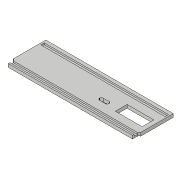
# Autodesk Inventor part: Electronics Container Part 4
Saved by Autodesk Inventor 2018.3 (Build 223284000, 284)
## iProperties
Created: 2019-03-04
Part Number: Electronics Container Part 4
Material: Generic
Document SubType Name: Modeling
Designer: aye06091
Mass: 12.6073 g
Surface Area: 108.421 cm^2
Volume: 12.6073 cm^3
Density: 1 g/cm^3
Appearance: Default
Author: aye06091
Autodesk Inventor part; units mm, degrees
ref_plane "YZ Plane" through (0, 0, 0) normal (1, 0, 0) x (0, 1, 0)
ref_plane "XZ Plane" through (0, 0, 0) normal (0, 1, 0) x (-1, 0, 0)
ref_plane "XY Plane" through (0, 0, 0) normal (0, 0, 1) x (1, 0, 0)
sketch "Sketch1" plane through (0, 0, 0) normal (0, 1, 0) x (-1, 0, 0)
  line L0 (0, 0) -> (-123.825, 0)
  line L1 (-123.825, 0) -> (-123.825, 38.1)
  line L2 (-123.825, 38.1) -> (0, 38.1)
  line L3 (0, 38.1) -> (0, 0)
  dimension "d0" = 123.825
  dimension "d1" = 38.1
  constraints: 8 end point, 2 parallel, 1 horizontal, 1 perpendicular
  measures "d0" distance of L0.start L0.end
  measures "d1" distance of L0.end L1.end
extrude "Extrusion1" add sketch "Sketch1" along normal blind 3.175
sketch "Sketch2" plane through (0, 3.175, 0) normal (0, 1, 0) x (1, 0, 0)
  line L0 (123.825, 0) -> (0, 0) projected
  line L1 (0, 0) -> (0, -38.1) projected
  line L2 (0, -38.1) -> (123.825, -38.1) projected
  line L3 (123.825, -38.1) -> (123.825, 0) projected
  line L4 (0, -36.5125) -> (123.825, -36.5125)
  line L5 (123.825, -36.5125) -> (123.825, -33.3121)
  line L6 (123.825, -33.3121) -> (0, -33.3121)
  line L7 (0, -33.3121) -> (0, -36.5125)
  line L8 (1.5875, -3.175) -> (122.2375, -3.175)
  line L9 (122.2375, -3.175) -> (122.2375, -6.604)
  line L10 (122.2375, -6.604) -> (1.5875, -6.604)
  line L11 (1.5875, -6.604) -> (1.5875, -3.175)
  dimension "d6" = 3.2004
  dimension "d7" = 1.5875
  dimension "d10" = 3.175
  dimension "d11" = 3.429
  dimension "d12" = 1.5875
  dimension "d13" = 1.5875
  constraints: 16 end point, 4 parallel, 2 horizontal, 2 perpendicular, 2 point on line
  measures "d6" distance between parallel lines of L4 L6
  measures "d7" distance between parallel lines of L2 L4
  measures "d10" distance between parallel lines of L0 L8
  measures "d11" distance between parallel lines of L10 L8
  measures "d12" distance between parallel lines of L1 L11
  measures "d13" distance between parallel lines of L3 L9
extrude "Extrusion2" cut sketch "Sketch2" against normal blind 1.5875 contours L3 L4 L1 L6
sketch "Sketch3" plane through (0, 3.175, 0) normal (0, 1, 0) x (1, 0, 0)
  line L0 (123.825, -33.3121) -> (123.825, 0) projected
  line L1 (123.825, 0) -> (0, 0) projected
  line L2 (0, 0) -> (0, -33.3121) projected
  line L3 (1.5875, -3.175) -> (122.2375, -3.175)
  line L4 (122.2375, -3.175) -> (122.2375, -6.604)
  line L5 (122.2375, -6.604) -> (1.5875, -6.604)
  line L6 (1.5875, -6.604) -> (1.5875, -3.175)
  dimension "d14" = 1.5875
  dimension "d15" = 1.5875
  dimension "d16" = 3.175
  dimension "d17" = 3.429
  constraints: 8 end point, 2 parallel, 1 horizontal, 1 perpendicular
  measures "d14" distance between parallel lines of L2 L6
  measures "d15" distance between parallel lines of L0 L4
  measures "d16" distance between parallel lines of L1 L3
  measures "d17" distance between parallel lines of L5 L3
extrude "Extrusion3" cut sketch "Sketch3" against normal blind 1.5875
sketch "Sketch4" plane through (0, 3.175, 0) normal (0, 1, 0) x (1, 0, 0)
  line L0 (0, -38.1) -> (1.5875, -38.1)
  line L1 (1.5875, -38.1) -> (1.5875, -31.75)
  line L2 (1.5875, -31.75) -> (0, -31.75)
  line L3 (0, -31.75) -> (0, -38.1)
  line L4 (123.825, -38.1) -> (122.2375, -38.1)
  line L5 (122.2375, -38.1) -> (122.2375, -31.75)
  line L6 (122.2375, -31.75) -> (123.825, -31.75)
  line L7 (123.825, -31.75) -> (123.825, -38.1)
  point P0 (0, 0)
  dimension "d20" = 1.5875
  dimension "d21" = 6.35
  dimension "d22" = 6.35
  dimension "d23" = 1.5875
  constraints: 16 end point, 4 parallel, 2 horizontal, 2 perpendicular
  measures "d20" distance of L1.end L2.end
  measures "d21" distance of L0.end L1.end
  measures "d22" distance of L4.end L5.end
  measures "d23" distance of L5.end L6.end
extrude "Extrusion4" cut sketch "Sketch4" against normal blind 25.4
fillet "Fillet1" radius 1.5875 1 edges at (122.2375, 1.5875, 31.75)
fillet "Fillet2" radius 1.5875 1 edges at (1.5875, 1.5875, 31.75)
sketch "Sketch5" plane through (0, 3.175, 0) normal (0, 1, 0) x (1, 0, 0)
  line L0 (1.5873, -33.3121) -> (122.2377, -33.3121) projected
  line L1 (74.9935, -21.0566) -> (84.1375, -21.0566)
  line L2 (84.1375, -21.0566) -> (84.1375, -24.6126)
  line L3 (84.1375, -24.6126) -> (74.9935, -24.6126)
  line L4 (74.9935, -24.6126) -> (74.9935, -21.0566)
  line L5 (122.2375, -36.5125) -> (122.2375, -33.3375) projected
  dimension "d28" = 8.6995
  dimension "d29" = 3.556
  dimension "d30" = 9.144
  dimension "d44" = 38.1
  constraints: 8 end point, 2 parallel, 1 horizontal, 1 perpendicular
  measures "d28" distance between parallel lines of L0 L3
  measures "d29" distance between parallel lines of L1 L3
  measures "d30" distance of L1.start L1.end
  measures "d44" distance between parallel lines of L5 L2
extrude "Extrusion5" cut sketch "Sketch5" against normal blind 25.4
fillet "Fillet3" radius 1.5875 4 edges at (74.9935, 1.5875, 21.0566) (84.1375, 1.5875, 21.0566) (84.1375, 1.5875, 24.6126) (74.9935, 1.5875, 24.6126)
sketch "Sketch6" plane through (0, 3.175, 0) normal (0, 1, 0) x (1, 0, 0)
  line L0 (1.5873, -33.3121) -> (122.2377, -33.3121) projected
  line L1 (93.6625, -14.7701) -> (119.6975, -14.7701)
  line L2 (119.6975, -14.7701) -> (119.6975, -26.2001)
  line L3 (119.6975, -26.2001) -> (93.6625, -26.2001)
  line L4 (93.6625, -26.2001) -> (93.6625, -14.7701)
  line L5 (122.2375, -36.5125) -> (122.2375, -33.3375) projected
  dimension "d35" = 26.035
  dimension "d36" = 11.43
  dimension "d41" = 7.112
  dimension "d43" = 2.54
  constraints: 8 end point, 2 parallel, 1 horizontal, 1 perpendicular
  measures "d35" distance of L1.start L1.end
  measures "d36" distance of L3.end L1.start
  measures "d41" distance between parallel lines of L0 L3
  measures "d43" distance between parallel lines of L5 L2
extrude "Extrusion6" cut sketch "Sketch6" against normal blind 25.4
body "Solid1"
